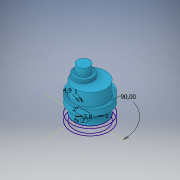
# Autodesk Inventor part: ExcentricShaft
Saved by Autodesk Inventor 2018.3 (Build 223284000, 284)
## iProperties
Created: 2018-07-20
Part Number: ExcentricShaft
Material: Generisch
Document SubType Name: Modeling
Designer: JochenAlt
Density: 1 g/cm^3
Appearance: Türkis
Author: JochenAlt
Autodesk Inventor part; units mm, degrees
ref_plane "YZ Plane" through (0, 0, 0) normal (1, 0, 0) x (0, 1, 0)
ref_plane "XZ Plane" through (0, 0, 0) normal (0, 1, 0) x (-1, 0, 0)
ref_plane "XY Plane" through (0, 0, 0) normal (0, 0, 1) x (1, 0, 0)
sketch "Skizze1" plane through (0, 0, 0) normal (0, 0, 1) x (1, 0, 0)
  line L0 (0, 14.0814) -> (0, -12.0814) construction
  line L1 (-12.0814, 0) -> (14.0814, 0) construction
  circle A0 centre (0, 0) radius 1.9
  arc A1 (-1.0971, -3.7971) -> (5.7971, 3.0971) centre (2, 0) ccw
  line L2 (0, -2) -> (0, 0) construction
  line L3 (0, 0) -> (2, 0) construction
  arc A2 (3.0971, 5.7971) -> (-3.7971, -1.0971) centre (0, 2) ccw
  arc A3 (-2.3174, -2.3174) -> (4.3174, 4.3174) centre (0, 2) ccw
  arc A4 (4.3174, 4.3174) -> (-2.3174, -2.3174) centre (2, 0) ccw
  line L4 (0, 0) -> (0, 8.4757) construction
  circle A5 centre (0, 0) radius 2.9
  arc A6 (5.0503, 5.0503) -> (3.0971, 5.7971) centre (2, 0) ccw
  arc A7 (5.7971, 3.0971) -> (4.3174, 4.3174) centre (2, 0) ccw
  arc A8 (3.0971, 5.7971) -> (-3.7971, -1.0971) centre (2, 0) ccw
  arc A9 (-3.0503, -3.0503) -> (5.0503, 5.0503) centre (2, 0) ccw
  arc A10 (-3.7971, -1.0971) -> (-3.0503, -3.0503) centre (2, 0) ccw
  arc A11 (-2.3174, -2.3174) -> (-1.0971, -3.7971) centre (2, 0) ccw
  arc A12 (-3.7971, -1.0971) -> (-2.3174, -2.3174) centre (0, 2) ccw
  arc A13 (-3.0503, -3.0503) -> (-1.0971, -3.7971) centre (0, 2) ccw
  arc A14 (-1.0971, -3.7971) -> (5.7971, 3.0971) centre (0, 2) ccw
  arc A15 (5.0503, 5.0503) -> (-3.0503, -3.0503) centre (0, 2) ccw
  arc A16 (4.3174, 4.3174) -> (3.0971, 5.7971) centre (0, 2) ccw
  arc A17 (5.7971, 3.0971) -> (5.0503, 5.0503) centre (0, 2) ccw
  dimension "d0" = 3.8
  dimension "d1" = 2
  dimension "d13" = 4.9
  dimension "d16" = 90
  dimension "d17" = 2
  dimension "d18" = 1
  dimension "d26" = 1
  constraints: 34 point on circle, 18 centre point, 14 equal radius, 6 end point, 4 coincident, 2 collinear, 2 concentric, 2 point on line, 1 perpendicular
  measures "d0" diameter of A0
  measures "d1" distance of point (0, 0) A2.centre
  measures "d13" radius of A2
  measures "d16" angle of L4 L1
  measures "d17" distance of point (0, 0) L3.end
  measures "d18" radial gap between concentric circles of A5 A0
  measures "d26" radial gap between concentric circles of A15 A2
extrude "Extrusion2" add sketch "Skizze1" along normal blind 4 contours A0 | A4 A5 A3 | A12 A8 A16 A4 | A3 A5 A4 | A5 | A2 A8
extrude "Extrusion8" add sketch "Skizze1" along normal blind 1 from surface at 4 contours A0 | A13 A10 A12 A11 | A11 A3 A7 A14 | A7 A16 A6 A17 | A4 A5 A3 | A12 A8 A16 A4 | A15 A6 A2 A10 | A3 A5 A4 | A5 | A2 A8
extrude "Extrusion3" add sketch "Skizze1" along normal blind 1 from surface at 5 contours A0 | A14 A1 | A13 A10 A12 A11 | A1 A17 A9 A13 | A11 A3 A7 A14 | A7 A16 A6 A17 | A4 A5 A3 | A12 A8 A16 A4 | A15 A6 A2 A10 | A3 A5 A4 | A5 | A2 A8
extrude "Extrusion9" add sketch "Skizze1" along normal blind 1 from surface at 6 contours A0 | A14 A1 | A13 A10 A12 A11 | A1 A17 A9 A13 | A11 A3 A7 A14 | A7 A16 A6 A17 | A4 A5 A3 | A12 A8 A16 A4 | A3 A5 A4 | A5
extrude "Extrusion4" add sketch "Skizze1" along normal blind 4 from surface at 7 contours A0 | A14 A1 | A11 A3 A7 A14 | A4 A5 A3 | A3 A5 A4 | A5
extrude "Extrusion7" add sketch "Skizze1" along normal blind 1 from surface at 11 contours A0 | A5
extrude "Extrusion5" add sketch "Skizze1" along normal blind 2.5 from surface at 12 contours A0
equation "\"d17\" = d1"
